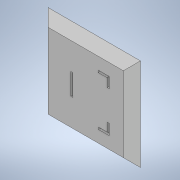
# Autodesk Inventor part: clear-square-outlined
Saved by Autodesk Inventor 2021 (Build 250183000, 183)
## iProperties
Created: 2020-12-08
Part Number: clear-square-outlined
Material: Generic
Document SubType Name: Modeling
Designer: Luke Kamols
Density: 1 g/cm^3
Appearance: Default
Author: Luke Kamols
Autodesk Inventor part; units mm, degrees
ref_plane "YZ Plane" through (0, 0, 0) normal (1, 0, 0) x (0, 1, 0)
ref_plane "XZ Plane" through (0, 0, 0) normal (0, 1, 0) x (-1, 0, 0)
ref_plane "XY Plane" through (0, 0, 0) normal (0, 0, 1) x (1, 0, 0)
sketch "Sketch1" plane through (0, 0, 0) normal (0, 0, 1) x (1, 0, 0)
  line L0 (0, 0) -> (43.2, 0)
  line L1 (43.2, 0) -> (43.2, 43.2)
  line L2 (43.2, 43.2) -> (0, 43.2)
  line L3 (0, 43.2) -> (0, 0)
  dimension "d0" = 43.2
  dimension "d1" = 43.2
  constraints: 8 end point, 2 parallel, 1 horizontal, 1 perpendicular
  measures "d0" distance of L2.end L1.end
  measures "d1" distance of L1.end L0.end
extrude "Extrusion1" add sketch "Sketch1" along normal blind 4
chamfer "Chamfer1" distance 4 angle 45 4 edges at (21.6, 43.2, 4) (43.2, 21.6, 4) (21.6, 0, 4) (0, 21.6, 4)
sketch "Sketch2" plane through (0, 0, 4) normal (0, 0, 1) x (1, 0, 0)
  line L0 (39.2, 4) -> (4, 4) projected
  line L1 (21.6, 4) -> (21.6, 39.2)
  line L2 (4, 39.2) -> (39.2, 39.2) projected
  line L3 (21.6, 39.2) -> (21.6, 38.6)
  line L4 (21.6, 38.6) -> (14.6, 38.6)
  line L5 (14.6, 38.6) -> (14.6, 4.6)
  line L6 (14.6, 4.6) -> (22.6, 4.6)
  line L7 (21.6, 38.6) -> (22.6, 38.6)
  line L8 (22.6, 38.6) -> (22.6, 33.6)
  line L9 (22.6, 33.6) -> (32.6, 33.6)
  line L10 (22.6, 4.6) -> (22.6, 9.6)
  line L11 (22.6, 9.6) -> (32.6, 9.6)
  line L12 (32.6, 9.6) -> (32.6, 33.6)
  line L13 (32.6, 33.6) -> (31.6, 33.6)
  line L14 (31.6, 32.6) -> (31.6, 28.6)
  line L15 (31.6, 28.6) -> (32.6, 28.6)
  line L16 (31.6, 32.6) -> (27.6, 32.6)
  line L17 (27.6, 32.6) -> (27.6, 33.6)
  line L18 (32.6, 9.6) -> (27.6, 9.6)
  line L19 (27.6, 9.6) -> (27.6, 10.6)
  line L20 (27.6, 10.6) -> (31.6, 10.6)
  line L21 (31.6, 10.6) -> (31.6, 14.6)
  line L22 (31.6, 14.6) -> (32.6, 14.6)
  line L23 (14.6, 21.6) -> (15.6, 21.6)
  line L24 (15.6, 21.6) -> (15.6, 26.6)
  line L25 (15.6, 26.6) -> (14.6, 26.6)
  line L26 (15.6, 21.6) -> (15.6, 16.6)
  line L27 (15.6, 16.6) -> (14.6, 16.6)
  point P0 (0, 0)
  dimension "d7" = 0.6
  dimension "d8" = 7
  dimension "d9" = 34
  dimension "d10" = 8
  dimension "d11" = 1
  dimension "d12" = 5
  dimension "d13" = 10
  dimension "d14" = 5
  dimension "d15" = 10
  dimension "d19" = 5
  dimension "d20" = 1
  dimension "d21" = 4
  dimension "d22" = 4
  dimension "d23" = 1
  dimension "d24" = 5
  dimension "d25" = 5
  constraints: 52 end point, 13 perpendicular, 6 point on line, 5 midpoint, 3 horizontal, 2 vertical, 1 parallel
  measures "d7" distance of L1.end L3.end
  measures "d8" distance of L3.end L4.end
  measures "d9" distance of L4.end L5.end
  measures "d10" distance of L5.end L6.end
  measures "d11" distance of L3.end L7.end
  measures "d12" distance of L7.end L8.end
  measures "d13" distance of L8.end L9.end
  measures "d14" distance of L6.end L10.end
  measures "d15" distance of L10.end L11.end
  measures "d19" distance of L11.end L18.end
  measures "d20" distance of L18.end L19.end
  measures "d21" distance of L19.end L20.end
  measures "d22" distance of L20.end L21.end
  measures "d23" distance of L23.start L23.end
  measures "d24" distance of L23.end L24.end
  measures "d25" distance of L23.end L26.end
extrude "Extrusion2" cut sketch "Sketch2" against normal blind 0.5 contours L5 L23 L26 L27 | L25 L24 L23 L5 | L19 L20 L21 L22 L12 L11 | L9 L12 L15 L14 L16 L17
chamfer "Chamfer2" distance 0.5 angle 45 6 edges at (27.6, 33.1, 3.5) (29.6, 32.6, 3.5) (31.6, 30.6, 3.5) (32.1, 28.6, 3.5) (32.6, 31.1, 3.5) (30.1, 33.6, 3.5)
chamfer "Chamfer3" distance 0.5 angle 45 10 edges at (27.6, 10.1, 3.5) (30.1, 9.6, 3.5) (31.6, 12.6, 3.5) (29.6, 10.6, 3.5) (32.1, 14.6, 3.5) (32.6, 12.1, 3.5) (15.1, 16.6, 3.5) (15.6, 21.6, 3.5) (15.1, 26.6, 3.5) (14.6, 21.6, 3.5)
body "Solid1"
